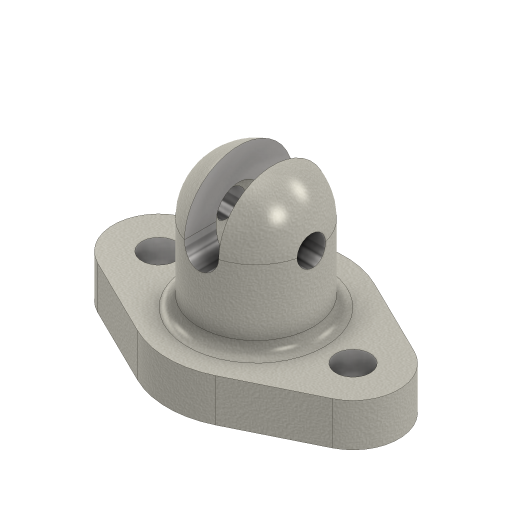
# Autodesk Inventor part: Part010TiltSupport
Saved by Autodesk Inventor 2023.2 (Build 272271030, 271C)
## iProperties
Created: 2023-09-11
Part Number: Part010TiltSupport
Material: Steel, Cast
Document SubType Name: Modeling
Designer: User
Mass: 696.896 g
Surface Area: 207.658 cm^2
Volume: 88.7766 cm^3
Density: 7.85 g/cm^3
Appearance: Steel - Cast
Author: User
Autodesk Inventor part; units mm, degrees
ref_plane "YZ Plane" through (0, 0, 0) normal (1, 0, 0) x (0, 1, 0)
ref_plane "XZ Plane" through (0, 0, 0) normal (0, 1, 0) x (-1, 0, 0)
ref_plane "XY Plane" through (0, 0, 0) normal (0, 0, 1) x (1, 0, 0)
sketch "Sketch1" plane through (0, 0, 0) normal (0, 1, 0) x (-1, 0, 0)
  line L0 (41.0588, -14.3587) -> (13.6765, -27.82)
  arc A0 (-13.6765, -27.82) -> (13.6765, -27.82) centre (0, 0) ccw
  line L1 (-13.6765, -27.82) -> (-41.0588, -14.3587)
  arc A1 (-41.0588, 14.3587) -> (-41.0588, -14.3587) centre (-34, 0) ccw
  line L2 (-41.0588, 14.3587) -> (-13.6765, 27.82)
  arc A2 (13.6765, 27.82) -> (-13.6765, 27.82) centre (0, 0) ccw
  line L3 (13.6765, 27.82) -> (41.0588, 14.3587)
  arc A3 (41.0588, -14.3587) -> (41.0588, 14.3587) centre (34, 0) ccw
  dimension "d0" = 68
  dimension "d1" = 16
  dimension "d2" = 31
  constraints: 8 end point, 8 point on circle, 7 tangent, 4 centre point, 2 coincident, 2 equal length, 2 equal radius, 2 horizontal alignment
  measures "d0" distance of A1.centre A3.centre
  measures "d1" radius of A1
  measures "d2" radius of A0
extrude "Extrusion1" add sketch "Sketch1" along normal blind 15
sketch "Sketch2" plane through (0, 15, 0) normal (0, 1, 0) x (1, 0, 0)
  arc A0 (-13.6765, -27.82) -> (13.6765, -27.82) centre (0, 0) ccw projected
  circle A1 centre (0, 0) radius 20
  dimension "d5" = 40
  constraints: 1 centre point, 1 coincident
  measures "d5" diameter of A1
extrude "Extrusion2" add sketch "Sketch2" along normal blind 27
fillet "Fillet1" radius 4 1 edges at (-20, 15, 0)
sketch "Sketch3" plane through (0, 0, 0) normal (0, 0, 1) x (1, 0, 0)
  line L0 (20, 42) -> (-20, 42) projected
  arc A0 (20, 42) -> (0, 62) centre (0, 42) ccw
  line L1 (0, -13.2284) -> (0, 79.3706) projected
  point P0 (0, 0)
  point P1 (0, 42)
  constraints: 2 point on circle, 1 centre point, 1 midpoint, 1 vertical alignment
revolve "Revolution1" add sketch "Sketch3" angle 360 about axis through (0, -10, 0) along (0, 1, 0)
sketch "Sketch4" plane through (0, 0, 0) normal (0, 0, 1) x (1, 0, 0)
  arc A0 (20, 42) -> (-20, 42) centre (0, 42) ccw projected
  arc A1 (20, 42) -> (-20, 42) centre (0, 42) ccw projected
  line L0 (10, 0) -> (10, 42)
  arc A2 (10, 42) -> (0, 52) centre (0, 42) ccw
  line L1 (0, -12.4) -> (0, 74.4) projected
  line L2 (10, 0) -> (0, 0)
  dimension "d10" = 20
  constraints: 4 end point, 2 point on circle, 1 centre point, 1 coincident, 1 horizontal, 1 tangent, 1 vertical, 1 vertical alignment
  measures "d10" diameter of L0 L1
revolve "Revolution2" cut sketch "Sketch4" angle 360 about axis through (0, -10, 0) along (0, 1, 0)
sketch "Sketch5" plane through (0, 0, 0) normal (0, 0, 1) x (1, 0, 0)
  arc A0 (10, 42) -> (-10, 42) centre (0, 42) ccw projected
  arc A1 (-6, 42) -> (6, 42) centre (0, 42) ccw
  line L0 (-6, 42) -> (-6, 61.0788)
  line L1 (6, 42) -> (6, 61.0788)
  line L2 (20, 42) -> (-20, 42) projected
  arc A2 (20, 42) -> (-20, 42) centre (0, 42) ccw projected
  arc A3 (6, 61.0788) -> (-6, 61.0788) centre (0, 42) ccw
  point P0 (0, 0)
  dimension "d12" = 6
  constraints: 6 point on circle, 4 end point, 2 centre point, 2 coincident, 2 point on line, 2 vertical
  measures "d12" radius of A1
extrude "Extrusion3" cut sketch "Sketch5" along normal through all both and the other way through all contours L1 L2 L0 A0 | A0 L0 A2 L1 | A1 L2
sketch "Sketch6" plane through (0, 0, 0) normal (1, 0, 0) x (0, 1, 0)
  arc A0 (42, -8) -> (42, 8) centre (42, 0) ccw projected
  circle A1 centre (42, 0) radius 5
  point P0 (0, 0)
  dimension "d15" = 10
  constraints: 1 centre point, 1 coincident
  measures "d15" diameter of A1
extrude "Extrusion4" cut sketch "Sketch6" along normal through all both and the other way through all
sketch "Sketch7" plane through (0, 15, 0) normal (0, 1, 0) x (1, 0, 0)
  arc A0 (41.0588, -14.3587) -> (41.0588, 14.3587) centre (34, 0) ccw projected
  arc A1 (-41.0588, 14.3587) -> (-41.0588, -14.3587) centre (-34, 0) ccw projected
hole "Hole1" at (-34, 15, 0) at (34, 15, 0) direction (0, -1, 0) diameter 12 end through all
body "Solid1"
